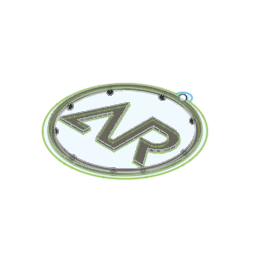
#AR_LLAVERO (Autodesk Fusion 360 design; units mm, degrees)
Autodesk Fusion 360 part; units mm, degrees
sketch "Boceto1" plane through (0, 0, 0) normal (0, 0, 1) x (1, 0, 0)
  spline S0 degree 3 poles (21.789, 0.8274) (20.982, 0.8754) (20.3216, 0.9315) (19.7996, 0.9964) knots 0 0 0 0 1 1 1 1
  spline S1 degree 3 poles (19.7996, 0.9964) (15.0608, 1.5857) (10.6601, 3.7164) (7.2118, 7.0912) knots 0 0 0 0 1 1 1 1
  spline S2 degree 3 poles (7.2118, 7.0912) (3.964, 10.2697) (1.7878, 14.3565) (0.9759, 18.8022) knots 0 0 0 0 1 1 1 1
  spline S3 degree 3 poles (0.9759, 18.8022) (0.732, 20.1376) (0.6241, 21.3519) (0.6241, 22.7633) knots 0 0 0 0 1 1 1 1
  spline S4 degree 3 poles (0.6241, 22.7633) (0.6241, 26.2437) (1.3989, 29.5188) (2.9549, 32.6162) knots 0 0 0 0 1 1 1 1
  spline S5 degree 3 poles (2.9549, 32.6162) (5.5283, 37.7387) (10.0589, 41.6898) (15.4644, 43.5253) knots 0 0 0 0 1 1 1 1
  spline S6 degree 3 poles (15.4644, 43.5253) (17.8229, 44.3262) (20.0704, 44.6977) (22.5585, 44.6977) knots 0 0 0 0 1 1 1 1
  spline S7 degree 3 poles (22.5585, 44.6977) (26.0418, 44.6977) (29.3112, 43.9243) (32.4114, 42.3669) knots 0 0 0 0 1 1 1 1
  spline S8 degree 3 poles (32.4114, 42.3669) (38.9324, 39.091) (43.4329, 32.7277) (44.3251, 25.5222) knots 0 0 0 0 1 1 1 1
  spline S9 degree 3 poles (44.3251, 25.5222) (44.4526, 24.4919) (44.4928, 23.8312) (44.4928, 22.7633) knots 0 0 0 0 1 1 1 1
  spline S10 degree 3 poles (44.4928, 22.7633) (44.4928, 18.8682) (43.516, 15.1989) (41.5823, 11.8303) knots 0 0 0 0 1 1 1 1
  spline S11 degree 3 poles (41.5823, 11.8303) (39.667, 8.4937) (36.8281, 5.6548) (33.4915, 3.7395) knots 0 0 0 0 1 1 1 1
  spline S12 degree 3 poles (33.4915, 3.7395) (30.6586, 2.1133) (27.6681, 1.1812) (24.3789, 0.8992) knots 0 0 0 0 1 1 1 1
  spline S13 degree 3 poles (24.3789, 0.8992) (23.7407, 0.8445) (22.2134, 0.8021) (21.789, 0.8274) knots 0 0 0 0 1 1 1 1
  spline S14 degree 3 poles (23.7971, 2.3085) (27.8943, 2.567) (31.6643, 3.956) (34.9293, 6.41) knots 0 0 0 0 1 1 1 1
  spline S15 degree 3 poles (34.9293, 6.41) (37.5968, 8.4149) (39.8339, 11.1933) (41.221, 14.2242) knots 0 0 0 0 1 1 1 1
  spline S16 degree 3 poles (41.221, 14.2242) (42.6211, 17.2831) (43.2576, 20.6913) (43.0498, 24.0151) knots 0 0 0 0 1 1 1 1
  spline S17 degree 3 poles (43.0498, 24.0151) (42.6813, 29.9078) (39.8585, 35.2883) (35.2265, 38.927) knots 0 0 0 0 1 1 1 1
  spline S18 degree 3 poles (35.2265, 38.927) (29.2563, 43.6169) (21.1453, 44.6099) (14.1882, 41.5027) knots 0 0 0 0 1 1 1 1
  spline S19 degree 3 poles (14.1882, 41.5027) (10.6334, 39.9151) (7.5143, 37.2423) (5.373, 33.9487) knots 0 0 0 0 1 1 1 1
  spline S20 degree 3 poles (5.373, 33.9487) (3.9151, 31.7064) (2.9221, 29.2263) (2.4241, 26.5833) knots 0 0 0 0 1 1 1 1
  spline S21 degree 3 poles (2.4241, 26.5833) (1.4455, 21.3905) (2.5011, 16.0327) (5.373, 11.6155) knots 0 0 0 0 1 1 1 1
  spline S22 degree 3 poles (5.373, 11.6155) (8.6676, 6.5481) (14.0271, 3.1853) (20.0012, 2.4372) knots 0 0 0 0 1 1 1 1
  spline S23 degree 3 poles (20.0012, 2.4372) (21.2873, 2.2762) (22.5863, 2.2321) (23.7971, 2.3085) knots 0 0 0 0 1 1 1 1
  spline S24 degree 3 poles (21.3949, 3.0617) (16.6195, 3.3312) (12.0641, 5.3754) (8.6499, 8.7812) knots 0 0 0 0 1 1 1 1
  spline S25 degree 3 poles (8.6499, 8.7812) (5.4692, 11.9541) (3.5115, 15.9535) (2.9665, 20.3925) knots 0 0 0 0 1 1 1 1
  spline S26 degree 3 poles (2.9665, 20.3925) (2.4077, 24.9428) (3.4557, 29.5365) (5.9434, 33.4409) knots 0 0 0 0 1 1 1 1
  spline S27 degree 3 poles (5.9434, 33.4409) (8.7014, 37.7697) (13.207, 40.9336) (18.2044, 42.0508) knots 0 0 0 0 1 1 1 1
  spline S28 degree 3 poles (18.2044, 42.0508) (23.0928, 43.1436) (28.2054, 42.3672) (32.4677, 39.8849) knots 0 0 0 0 1 1 1 1
  spline S29 degree 3 poles (32.4677, 39.8849) (37.2437, 37.1033) (40.658, 32.4687) (41.8459, 27.1549) knots 0 0 0 0 1 1 1 1
  spline S30 degree 3 poles (41.8459, 27.1549) (42.9393, 22.264) (42.1687, 17.1878) (39.6807, 12.8917) knots 0 0 0 0 1 1 1 1
  spline S31 degree 3 poles (39.6807, 12.8917) (38.2703, 10.4562) (36.3242, 8.3167) (34.0414, 6.6919) knots 0 0 0 0 1 1 1 1
  spline S32 degree 3 poles (34.0414, 6.6919) (30.35, 4.0645) (25.9594, 2.8042) (21.3949, 3.0617) knots 0 0 0 0 1 1 1 1
  line L0 (15.5394, 15.3443) -> (15.5394, 16.6333)
  line L1 (15.5394, 16.6333) -> (13.2088, 16.6552)
  spline S33 degree 3 poles (13.2088, 16.6552) (11.9269, 16.6673) (10.8693, 16.686) (10.8586, 16.6967) knots 0 0 0 0 1 1 1 1
  spline S34 degree 3 poles (10.8586, 16.6967) (10.8398, 16.7155) (11.0307, 17.1566) (11.6564, 18.5407) knots 0 0 0 0 1 1 1 1
  spline S35 degree 3 poles (11.6564, 18.5407) (11.9273, 19.1399) (12.0928, 19.5085) (12.6674, 20.7928) knots 0 0 0 0 1 1 1 1
  spline S36 degree 3 poles (12.6674, 20.7928) (12.7968, 21.0818) (13.0125, 21.5632) (13.1469, 21.8625) knots 0 0 0 0 1 1 1 1
  spline S37 degree 3 poles (13.1469, 21.8625) (13.2813, 22.1618) (13.5391, 22.7361) (13.7197, 23.1387) knots 0 0 0 0 1 1 1 1
  spline S38 degree 3 poles (13.7197, 23.1387) (13.9004, 23.5412) (14.1738, 24.1493) (14.3274, 24.4899) knots 0 0 0 0 1 1 1 1
  spline S39 degree 3 poles (14.3274, 24.4899) (14.4809, 24.8306) (14.6847, 25.2845) (14.7802, 25.4988) knots 0 0 0 0 1 1 1 1
  line L2 (14.7802, 25.4988) -> (14.9539, 25.8883)
  line L3 (14.9539, 25.8883) -> (15.0818, 25.6114)
  spline S40 degree 3 poles (15.0818, 25.6114) (15.1522, 25.4591) (15.3161, 25.098) (15.4459, 24.809) knots 0 0 0 0 1 1 1 1
  spline S41 degree 3 poles (15.4459, 24.809) (15.7368, 24.1617) (16.121, 23.3091) (16.4735, 22.5287) knots 0 0 0 0 1 1 1 1
  spline S42 degree 3 poles (16.4735, 22.5287) (16.6204, 22.2036) (16.8588, 21.6758) (17.0033, 21.3558) knots 0 0 0 0 1 1 1 1
  spline S43 degree 3 poles (17.0033, 21.3558) (17.1478, 21.0358) (17.3843, 20.5122) (17.5288, 20.1922) knots 0 0 0 0 1 1 1 1
  spline S44 degree 3 poles (17.5288, 20.1922) (17.6733, 19.8722) (17.9098, 19.3486) (18.0543, 19.0286) knots 0 0 0 0 1 1 1 1
  spline S45 degree 3 poles (18.0543, 19.0286) (18.1988, 18.7086) (18.4373, 18.1808) (18.5843, 17.8557) knots 0 0 0 0 1 1 1 1
  spline S46 degree 3 poles (18.5843, 17.8557) (18.7312, 17.5305) (18.9577, 17.028) (19.0876, 16.739) knots 0 0 0 0 1 1 1 1
  spline S47 degree 3 poles (19.0876, 16.739) (19.2175, 16.45) (19.4536, 15.9264) (19.6123, 15.5754) knots 0 0 0 0 1 1 1 1
  spline S48 degree 3 poles (19.6123, 15.5754) (19.7711, 15.2245) (19.9764, 14.7684) (20.0686, 14.562) knots 0 0 0 0 1 1 1 1
  spline S49 degree 3 poles (20.0686, 14.562) (20.1608, 14.3555) (20.2637, 14.1655) (20.2973, 14.1397) knots 0 0 0 0 1 1 1 1
  spline S50 degree 3 poles (20.2973, 14.1397) (20.377, 14.0784) (26.9134, 14.0705) (27.0275, 14.1316) knots 0 0 0 0 1 1 1 1
  spline S51 degree 3 poles (27.0275, 14.1316) (27.0989, 14.1698) (27.1001, 14.2919) (27.1, 21.4167) knots 0 0 0 0 1 1 1 1
  spline S52 degree 3 poles (27.1, 21.4167) (27.0999, 28.2025) (27.1039, 28.6699) (27.1644, 28.7722) knots 0 0 0 0 1 1 1 1
  line L4 (27.1644, 28.7722) -> (27.229, 28.8815)
  line L5 (27.229, 28.8815) -> (29.5762, 28.8809)
  spline S53 degree 3 poles (29.5762, 28.8809) (32.1767, 28.8802) (32.2205, 28.8768) (32.7177, 28.6407) knots 0 0 0 0 1 1 1 1
  spline S54 degree 3 poles (32.7177, 28.6407) (33.1079, 28.4554) (33.3913, 28.2517) (33.6692, 27.9569) knots 0 0 0 0 1 1 1 1
  spline S55 degree 3 poles (33.6692, 27.9569) (34.3728, 27.2103) (34.6361, 26.2136) (34.3955, 25.207) knots 0 0 0 0 1 1 1 1
  spline S56 degree 3 poles (34.3955, 25.207) (34.3639, 25.0749) (34.3248, 24.9398) (34.3086, 24.9067) knots 0 0 0 0 1 1 1 1
  spline S57 degree 3 poles (34.3086, 24.9067) (34.2924, 24.8736) (34.2424, 24.7705) (34.1976, 24.6776) knots 0 0 0 0 1 1 1 1
  spline S58 degree 3 poles (34.1976, 24.6776) (34.0826, 24.4395) (34.034, 24.3597) (33.9194, 24.2214) knots 0 0 0 0 1 1 1 1
  spline S59 degree 3 poles (33.9194, 24.2214) (33.8641, 24.1547) (33.8189, 24.0858) (33.8189, 24.0682) knots 0 0 0 0 1 1 1 1
  spline S60 degree 3 poles (33.8189, 24.0682) (33.8189, 24.0164) (33.5586, 23.7502) (33.3528, 23.5916) knots 0 0 0 0 1 1 1 1
  spline S61 degree 3 poles (33.3528, 23.5916) (33.1666, 23.4481) (32.6018, 23.1389) (32.525, 23.1385) knots 0 0 0 0 1 1 1 1
  spline S62 degree 3 poles (32.525, 23.1385) (32.5038, 23.1383) (32.4358, 23.1116) (32.3738, 23.0791) knots 0 0 0 0 1 1 1 1
  spline S63 degree 3 poles (32.3738, 23.0791) (32.1091, 22.9401) (31.7231, 22.9136) (29.9622, 22.9135) knots 0 0 0 0 1 1 1 1
  spline S64 degree 3 poles (29.9622, 22.9135) (29.0281, 22.9135) (28.2638, 22.9036) (28.2638, 22.8916) knots 0 0 0 0 1 1 1 1
  spline S65 degree 3 poles (28.2638, 22.8916) (28.2638, 22.8695) (29.3359, 21.318) (29.5195, 21.0743) knots 0 0 0 0 1 1 1 1
  spline S66 degree 3 poles (29.5195, 21.0743) (29.574, 21.002) (29.9328, 20.4869) (30.3169, 19.9295) knots 0 0 0 0 1 1 1 1
  spline S67 degree 3 poles (30.3169, 19.9295) (30.7009, 19.3721) (31.1507, 18.7218) (31.3163, 18.4844) knots 0 0 0 0 1 1 1 1
  spline S68 degree 3 poles (31.3163, 18.4844) (31.5664, 18.126) (31.9075, 17.6338) (33.1809, 15.7945) knots 0 0 0 0 1 1 1 1
  spline S69 degree 3 poles (33.1809, 15.7945) (33.2118, 15.7499) (33.3895, 15.4965) (33.5758, 15.2315) knots 0 0 0 0 1 1 1 1
  spline S70 degree 3 poles (33.5758, 15.2315) (34.0797, 14.5144) (34.2083, 14.3265) (34.2581, 14.2346) knots 0 0 0 0 1 1 1 1
  spline S71 degree 3 poles (34.2581, 14.2346) (34.283, 14.1888) (34.3336, 14.1392) (34.3707, 14.1243) knots 0 0 0 0 1 1 1 1
  spline S72 degree 3 poles (34.3707, 14.1243) (34.4481, 14.0933) (37.5265, 14.089) (37.7163, 14.1196) knots 0 0 0 0 1 1 1 1
  spline S73 degree 3 poles (37.7163, 14.1196) (37.8104, 14.1348) (37.8373, 14.1555) (37.8248, 14.2032) knots 0 0 0 0 1 1 1 1
  spline S74 degree 3 poles (37.8248, 14.2032) (37.8087, 14.2651) (37.3956, 14.8501) (35.9916, 16.8002) knots 0 0 0 0 1 1 1 1
  spline S75 degree 3 poles (35.9916, 16.8002) (33.6607, 20.0374) (33.2895, 20.5576) (33.3022, 20.5692) knots 0 0 0 0 1 1 1 1
  spline S76 degree 3 poles (33.3022, 20.5692) (33.3077, 20.5742) (33.4727, 20.6317) (33.6688, 20.6968) knots 0 0 0 0 1 1 1 1
  spline S77 degree 3 poles (33.6688, 20.6968) (34.0257, 20.8153) (34.7419, 21.1511) (34.9751, 21.3092) knots 0 0 0 0 1 1 1 1
  spline S78 degree 3 poles (34.9751, 21.3092) (35.0433, 21.3555) (35.1859, 21.4651) (35.2919, 21.5528) knots 0 0 0 0 1 1 1 1
  spline S79 degree 3 poles (35.2919, 21.5528) (35.398, 21.6406) (35.496, 21.7124) (35.5098, 21.7124) knots 0 0 0 0 1 1 1 1
  spline S80 degree 3 poles (35.5098, 21.7124) (35.5534, 21.7124) (36.1144, 22.2807) (36.21, 22.4217) knots 0 0 0 0 1 1 1 1
  spline S81 degree 3 poles (36.21, 22.4217) (36.2604, 22.4961) (36.3515, 22.6118) (36.4124, 22.6789) knots 0 0 0 0 1 1 1 1
  spline S82 degree 3 poles (36.4124, 22.6789) (36.4734, 22.746) (36.54, 22.8389) (36.5604, 22.8854) knots 0 0 0 0 1 1 1 1
  spline S83 degree 3 poles (36.5604, 22.8854) (36.5808, 22.9318) (36.6334, 23.0289) (36.6773, 23.1012) knots 0 0 0 0 1 1 1 1
  spline S84 degree 3 poles (36.6773, 23.1012) (37.0047, 23.6397) (37.2848, 24.3809) (37.4079, 25.0342) knots 0 0 0 0 1 1 1 1
  spline S85 degree 3 poles (37.4079, 25.0342) (37.5021, 25.5345) (37.5022, 26.6965) (37.4081, 27.1174) knots 0 0 0 0 1 1 1 1
  spline S86 degree 3 poles (37.4081, 27.1174) (37.2502, 27.8233) (36.8994, 28.7437) (36.6572, 29.0875) knots 0 0 0 0 1 1 1 1
  spline S87 degree 3 poles (36.6572, 29.0875) (36.6134, 29.1497) (36.5607, 29.228) (36.5401, 29.2614) knots 0 0 0 0 1 1 1 1
  spline S88 degree 3 poles (36.5401, 29.2614) (36.3596, 29.5549) (35.504, 30.4944) (35.4166, 30.4952) knots 0 0 0 0 1 1 1 1
  spline S89 degree 3 poles (35.4166, 30.4952) (35.3973, 30.4954) (35.3044, 30.5597) (35.2101, 30.6381) knots 0 0 0 0 1 1 1 1
  spline S90 degree 3 poles (35.2101, 30.6381) (35.021, 30.7955) (34.7979, 30.9312) (34.4007, 31.1306) knots 0 0 0 0 1 1 1 1
  spline S91 degree 3 poles (34.4007, 31.1306) (33.9381, 31.3629) (33.4782, 31.5101) (32.8243, 31.6353) knots 0 0 0 0 1 1 1 1
  line L6 (32.8243, 31.6353) -> (32.3738, 31.7215)
  line L7 (32.3738, 31.7215) -> (28.2168, 31.7052)
  line L8 (28.2168, 31.7052) -> (24.0599, 31.6889)
  line L9 (24.0599, 31.6889) -> (24.0599, 24.2255)
  spline S92 degree 3 poles (24.0599, 24.2255) (24.0599, 20.1207) (24.0472, 16.7547) (24.0317, 16.7456) knots 0 0 0 0 1 1 1 1
  spline S93 degree 3 poles (24.0317, 16.7456) (23.9752, 16.7124) (22.2207, 16.7688) (22.2207, 16.8039) knots 0 0 0 0 1 1 1 1
  spline S94 degree 3 poles (22.2207, 16.8039) (22.2207, 16.8234) (22.062, 17.163) (21.8682, 17.5586) knots 0 0 0 0 1 1 1 1
  spline S95 degree 3 poles (21.8682, 17.5586) (21.5509, 18.206) (21.3441, 18.6363) (20.963, 19.4415) knots 0 0 0 0 1 1 1 1
  spline S96 degree 3 poles (20.963, 19.4415) (20.8946, 19.586) (20.7001, 19.9914) (20.5307, 20.3423) knots 0 0 0 0 1 1 1 1
  spline S97 degree 3 poles (20.5307, 20.3423) (20.3613, 20.6933) (20.0999, 21.2422) (19.9497, 21.5622) knots 0 0 0 0 1 1 1 1
  spline S98 degree 3 poles (19.9497, 21.5622) (19.7995, 21.8822) (19.5713, 22.3636) (19.4426, 22.632) knots 0 0 0 0 1 1 1 1
  spline S99 degree 3 poles (19.4426, 22.632) (19.1541, 23.2336) (18.9232, 23.7246) (18.7895, 24.0208) knots 0 0 0 0 1 1 1 1
  spline S100 degree 3 poles (18.7895, 24.0208) (18.7335, 24.1446) (18.6719, 24.2713) (18.6525, 24.3023) knots 0 0 0 0 1 1 1 1
  spline S101 degree 3 poles (18.6525, 24.3023) (18.633, 24.3332) (18.6017, 24.3938) (18.583, 24.4368) knots 0 0 0 0 1 1 1 1
  spline S102 degree 3 poles (18.583, 24.4368) (18.5642, 24.4799) (18.4269, 24.767) (18.278, 25.0749) knots 0 0 0 0 1 1 1 1
  spline S103 degree 3 poles (18.278, 25.0749) (18.129, 25.3828) (17.9408, 25.7783) (17.8598, 25.9538) knots 0 0 0 0 1 1 1 1
  spline S104 degree 3 poles (17.8598, 25.9538) (17.7787, 26.1293) (17.6462, 26.408) (17.5653, 26.5731) knots 0 0 0 0 1 1 1 1
  spline S105 degree 3 poles (17.5653, 26.5731) (17.2941, 27.1269) (16.7721, 28.2144) (16.6211, 28.5402) knots 0 0 0 0 1 1 1 1
  spline S106 degree 3 poles (16.6211, 28.5402) (16.5388, 28.7176) (16.2299, 29.3695) (15.9347, 29.9888) knots 0 0 0 0 1 1 1 1
  spline S107 degree 3 poles (15.9347, 29.9888) (15.289, 31.3431) (15.1087, 31.7251) (14.9869, 31.9964) knots 0 0 0 0 1 1 1 1
  spline S108 degree 3 poles (14.9869, 31.9964) (14.9004, 32.1891) (14.8911, 32.1976) (14.8416, 32.1299) knots 0 0 0 0 1 1 1 1
  spline S109 degree 3 poles (14.8416, 32.1299) (14.8125, 32.0902) (14.7887, 32.0376) (14.7887, 32.013) knots 0 0 0 0 1 1 1 1
  spline S110 degree 3 poles (14.7887, 32.013) (14.7887, 31.9735) (14.5605, 31.4783) (13.5879, 29.407) knots 0 0 0 0 1 1 1 1
  spline S111 degree 3 poles (13.5879, 29.407) (13.1765, 28.5309) (12.753, 27.6267) (12.4803, 27.0423) knots 0 0 0 0 1 1 1 1
  spline S112 degree 3 poles (12.4803, 27.0423) (12.3407, 26.743) (12.0954, 26.2194) (11.9352, 25.8787) knots 0 0 0 0 1 1 1 1
  spline S113 degree 3 poles (11.9352, 25.8787) (11.775, 25.5381) (11.4541, 24.854) (11.2222, 24.3586) knots 0 0 0 0 1 1 1 1
  spline S114 degree 3 poles (11.2222, 24.3586) (10.1283, 22.0222) (9.6182, 20.9338) (9.3661, 20.3986) knots 0 0 0 0 1 1 1 1
  spline S115 degree 3 poles (9.3661, 20.3986) (9.0885, 19.8093) (8.7968, 19.1868) (8.28, 18.0809) knots 0 0 0 0 1 1 1 1
  spline S116 degree 3 poles (8.28, 18.0809) (8.1232, 17.7454) (7.8667, 17.1964) (7.7099, 16.861) knots 0 0 0 0 1 1 1 1
  spline S117 degree 3 poles (7.7099, 16.861) (7.0723, 15.4966) (6.5362, 14.3691) (6.3892, 14.0834) knots 0 0 0 0 1 1 1 1
  spline S118 degree 3 poles (6.3892, 14.0834) (6.3812, 14.0679) (8.4367, 14.0552) (10.9571, 14.0552) knots 0 0 0 0 1 1 1 1
  line L10 (10.9571, 14.0552) -> (15.5394, 14.0552)
  line L11 (15.5394, 14.0552) -> (15.5394, 15.3443)
  circle A0 centre (22.5585, 44.524) radius 1.25
  arc A1 (25.0582, 44.5608) -> (20.0588, 44.5631) centre (22.5585, 44.524) ccw
  spline S119 degree 3 poles (31.9644, 39.0208) (36.5021, 36.378) (39.7441, 31.9732) (40.87, 26.9368) knots 0 0 0 0 1 1 1 1
  spline S120 degree 3 poles (40.87, 26.9368) (41.9094, 22.2872) (41.177, 17.4708) (38.8154, 13.3928) knots 0 0 0 0 1 1 1 1
  spline S121 degree 3 poles (38.8154, 13.3928) (37.4776, 11.0828) (35.6252, 9.0466) (33.4615, 7.5066) knots 0 0 0 0 1 1 1 1
  spline S122 degree 3 poles (33.4615, 7.5066) (29.9522, 5.0088) (25.7965, 3.815) (21.4512, 4.0602) knots 0 0 0 0 1 1 1 1
  spline S123 degree 3 poles (21.4512, 4.0602) (16.9241, 4.3156) (12.5971, 6.2562) (9.3562, 9.4891) knots 0 0 0 0 1 1 1 1
  spline S124 degree 3 poles (9.3562, 9.4891) (6.3276, 12.5102) (4.4776, 16.2907) (3.959, 20.5143) knots 0 0 0 0 1 1 1 1
  spline S125 degree 3 poles (3.959, 20.5143) (3.4286, 24.8338) (4.4217, 29.1915) (6.7867, 32.9035) knots 0 0 0 0 1 1 1 1
  spline S126 degree 3 poles (6.7867, 32.9035) (9.3982, 37.0024) (13.6925, 40.0175) (18.4226, 41.0749) knots 0 0 0 0 1 1 1 1
  spline S127 degree 3 poles (18.4226, 41.0749) (23.0677, 42.1133) (27.9243, 41.3737) (31.9644, 39.0208) knots 0 0 0 0 1 1 1 1
  dimension "d1" = 5
  dimension "d2" = 2.5
  dimension "d13" = 1
  constraint concentric A0 A1
  constraint coincident S7 A1.start
  constraint coincident S6 A1.end
  measures "d1" diameter of A1
  measures "d2" diameter of A0
extrude "Extruir1" add sketch "Boceto1" along normal blind 1.5 contours S0 S1 S2 S3 S4 S5 S6 S7 S8 S9 S10 S11 S12 S13 S14 S15 S16 S17 S18 S19 S20 S21 S22 S23 A0 | S6 S7 A0 A1 | S24 S25 S26 S27 S28 S29 S30 S31 S32 | S119 S120 S121 S122 S123 S124 S125 S126 S127 makes body 1 at (5.8656, 10.135, 0) makes body 2 at (19.0837, 35.2454, 0)
extrude "Extruir2" add sketch "Boceto1" along normal blind 0.25 contours S14 S15 S16 S17 S18 S19 S20 S21 S22 S23 A0 | S24 S25 S26 S27 S28 S29 S30 S31 S32 | L0 L1 S33 S34 S35 S36 S37 S38 S39 L2 L3 S40 S41 S42 S43 S44 S45 S46 S47 S48 S49 S50 S51 S52 L4 L5 S53 S54 S55 S56 S57 S58 S59 S60 S61 S62 S63 S64 S65 S66 S67 S68 S69 S70 S71 S72 S73 S74 S75 S76 S77 S78 S79 S80 S81 S82 S83 S84 S85 S86 S87 S88 S89 S90 S91 L6 L7 L8 L9 S92 S93 S94 S95 S96 S97 S98 S99 S100 S101 S102 S103 S104 S105 S106 S107 S108 S109 S110 S111 S112 S113 S114 S115 S116 S117 S118 L10 L11 | S119 S120 S121 S122 S123 S124 S125 S126 S127 bodies 2 1
extrude "Extruir4" add sketch "Boceto1" along normal blind 1 separate body contours S14 S15 S16 S17 S18 S19 S20 S21 S22 S23 A0 | S24 S25 S26 S27 S28 S29 S30 S31 S32 | L0 L1 S33 S34 S35 S36 S37 S38 S39 L2 L3 S40 S41 S42 S43 S44 S45 S46 S47 S48 S49 S50 S51 S52 L4 L5 S53 S54 S55 S56 S57 S58 S59 S60 S61 S62 S63 S64 S65 S66 S67 S68 S69 S70 S71 S72 S73 S74 S75 S76 S77 S78 S79 S80 S81 S82 S83 S84 S85 S86 S87 S88 S89 S90 S91 L6 L7 L8 L9 S92 S93 S94 S95 S96 S97 S98 S99 S100 S101 S102 S103 S104 S105 S106 S107 S108 S109 S110 S111 S112 S113 S114 S115 S116 S117 S118 L10 L11 makes body 3 at (8.0272, 10.098, 0) makes body 4 at (25.0764, 27.8384, 0)
hidden bodies 2
named bodies: "LL_AR"
